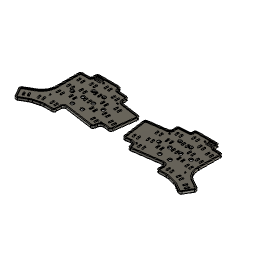
MUSUBI_V2_CASE (Autodesk Fusion 360 design; units mm, degrees)
Autodesk Fusion 360 part; units mm, degrees
note: some values were not read from the file. Set by a fixed rule: which sketch regions a step uses.
sketch "WIP_rev2_case" plane through (0, 0, 0) normal (0, 0, 1) x (1, 0, 0)
  line L0 (119.3956, 43.1697) -> (120.5503, 41.1697)
  line L1 (12.5668, 44.6925) -> (7.0696, 83.8079)
  arc A0 (148.5082, 9.578) -> (145.7761, 8.8459) centre (146.7761, 10.578) cw
  arc A1 (104.7713, 110.126) -> (104.7713, 112.726) centre (104.7713, 111.426) ccw
  line L2 (8.7718, 86.0667) -> (41.7893, 90.7069)
  line L3 (96.0593, 110.126) -> (104.7713, 110.126)
  line L4 (87.3832, 39.0506) -> (35.5891, 31.7716)
  circle A2 centre (69.0928, 67.7697) radius 20.55
  arc A3 (35.5891, 31.7716) -> (33.3302, 33.4738) centre (35.3107, 33.7521) cw
  arc A4 (41.7893, 90.7069) -> (46.9396, 97.0671) centre (40.9543, 96.6485) ccw
  arc A5 (46.5363, 102.8343) -> (48.392, 104.969) centre (48.5315, 102.9738) cw
  line L5 (30.8499, 43.0697) -> (33.1593, 43.0697)
  line L6 (93.8874, 109.0668) -> (92.7327, 111.0668)
  line L7 (90.4233, 107.0668) -> (92.7327, 107.0668)
  line L8 (92.7327, 107.0668) -> (93.8874, 109.0668)
  line L9 (145.7761, 8.8459) -> (133.5777, 15.8887)
  arc A6 (14.8256, 42.9903) -> (12.5668, 44.6925) centre (14.5473, 44.9709) cw
  line L10 (120.5503, 45.1697) -> (119.3956, 43.1697)
  line L11 (48.392, 104.969) -> (64.952, 106.127)
  line L12 (68.673, 110.1172) -> (68.673, 112.1248)
  line L13 (45.7503, 91.2697) -> (44.5956, 89.2697)
  line L14 (107.673, 112.1248) -> (107.673, 106.1248)
  line L15 (70.673, 114.1248) -> (105.673, 114.1248)
  arc A7 (156.0261, 26.5995) -> (156.7582, 23.8674) centre (155.0261, 24.8674) cw
  arc A8 (68.673, 112.1248) -> (70.673, 114.1248) centre (70.673, 112.1248) cw
  line L16 (46.9396, 97.0671) -> (46.5363, 102.8343)
  arc A9 (133.5777, 15.8887) -> (127.7892, 18.2864) centre (121.5777, -4.8959) ccw
  arc A10 (107.673, 106.1248) -> (111.673, 102.1248) centre (111.673, 106.1248) ccw
  line L17 (111.673, 102.1248) -> (124.173, 102.1248)
  arc A11 (96.0593, 105.5236) -> (96.0593, 108.1236) centre (96.0593, 106.8236) cw
  arc A12 (126.173, 60.001) -> (140.173, 35.7523) centre (154.173, 60.001) ccw
  arc A13 (124.173, 102.1248) -> (126.173, 100.1248) centre (124.173, 100.1248) cw
  line L18 (156.7582, 23.8674) -> (148.5082, 9.578)
  circle A14 centre (32.0046, 45.0697) radius 1.3
  line L19 (89.2686, 109.0668) -> (90.4233, 107.0668)
  arc A15 (32.7737, 37.4339) -> (23.7383, 44.2427) centre (24.8515, 36.3206) ccw
  circle A16 centre (106.9188, 67.9606) radius 3.2
  arc A17 (104.7713, 108.1236) -> (104.7713, 105.5236) centre (104.7713, 106.8236) cw
  line L20 (122.8597, 41.1697) -> (124.0144, 43.1697)
  line L21 (33.1593, 47.0697) -> (30.8499, 47.0697)
  circle A18 centre (50.0544, 67.1169) radius 3.2
  arc A19 (7.0696, 83.8079) -> (8.7718, 86.0667) centre (9.0501, 84.0862) cw
  circle A20 centre (91.578, 109.0668) radius 1.3
  arc A21 (105.673, 114.1248) -> (107.673, 112.1248) centre (105.673, 112.1248) cw
  circle A22 centre (69.7456, 48.7314) radius 3.2
  arc A23 (96.2183, 22.1248) -> (94.2183, 24.1248) centre (96.2183, 24.1248) cw
  line L22 (126.173, 100.1248) -> (126.173, 60.001)
  line L23 (49.2144, 89.2697) -> (48.0597, 91.2697)
  line L24 (92.7327, 111.0668) -> (90.4233, 111.0668)
  circle A24 centre (68.8188, 67.9849) radius 3.2
  line L25 (122.8597, 45.1697) -> (120.5503, 45.1697)
  line L26 (90.4233, 111.0668) -> (89.2686, 109.0668)
  line L27 (104.7713, 112.726) -> (96.0593, 112.726)
  line L28 (34.314, 45.0697) -> (33.1593, 47.0697)
  line L29 (45.7503, 87.2697) -> (48.0597, 87.2697)
  arc A25 (94.2183, 33.109) -> (87.3832, 39.0506) centre (88.2183, 33.109) ccw
  line L30 (23.7383, 44.2427) -> (14.8256, 42.9903)
  line L31 (29.6952, 45.0697) -> (30.8499, 43.0697)
  line L32 (48.0597, 91.2697) -> (45.7503, 91.2697)
  circle A26 centre (87.8567, 48.9227) radius 3.2
  line L33 (33.1593, 43.0697) -> (34.314, 45.0697)
  circle A27 centre (88.1311, 68.4225) radius 3.2
  circle A28 centre (87.881, 87.0227) radius 3.2
  line L34 (30.8499, 47.0697) -> (29.6952, 45.0697)
  line L35 (48.0597, 87.2697) -> (49.2144, 89.2697)
  line L36 (33.3302, 33.4738) -> (32.7737, 37.4339)
  line L37 (110.304, 22.1248) -> (96.2183, 22.1248)
  line L38 (120.5503, 41.1697) -> (122.8597, 41.1697)
  circle A29 centre (46.905, 89.2697) radius 1.3
  circle A30 centre (121.705, 43.1697) radius 1.3
  circle A31 centre (87.8688, 67.9727) radius 20.55
  circle A32 centre (68.44, 86.8081) radius 3.2
  line L39 (96.0593, 108.1236) -> (104.7713, 108.1236)
  line L40 (104.7713, 105.5236) -> (96.0593, 105.5236)
  arc A33 (96.0593, 112.726) -> (96.0593, 110.126) centre (96.0593, 111.426) ccw
  arc A34 (64.952, 106.127) -> (68.673, 110.1172) centre (64.673, 110.1172) ccw
  line L41 (140.173, 35.7523) -> (156.0261, 26.5995)
  line L42 (44.5956, 89.2697) -> (45.7503, 87.2697)
  line L43 (124.0144, 43.1697) -> (122.8597, 45.1697)
  arc A35 (116.5155, 21.3071) -> (110.304, 22.1248) centre (110.304, -1.8752) ccw
  line L44 (127.7892, 18.2864) -> (116.5155, 21.3071)
  line L45 (87.6616, 37.0701) -> (35.8674, 29.791)
  arc A36 (30.7931, 37.1556) -> (24.0166, 42.2622) centre (24.8515, 36.3206) ccw
  arc A37 (35.8674, 29.791) -> (31.3497, 33.1954) centre (35.3107, 33.7521) cw
  line L46 (94.2183, 24.1248) -> (94.2183, 33.109)
  arc A38 (92.2183, 33.109) -> (87.6616, 37.0701) centre (88.2183, 33.109) ccw
  line L47 (31.3497, 33.1954) -> (30.7931, 37.1556)
  line L48 (24.0166, 42.2622) -> (15.1039, 41.0098)
  arc A39 (15.1039, 41.0098) -> (10.5862, 44.4142) centre (14.5473, 44.9709) cw
  arc A40 (105.673, 116.1248) -> (109.673, 112.1248) centre (105.673, 112.1248) cw
  arc A41 (64.8125, 108.1221) -> (66.673, 110.1172) centre (64.673, 110.1172) ccw
  line L49 (44.9445, 96.9276) -> (44.5412, 102.6948)
  line L50 (109.673, 112.1248) -> (109.673, 106.1248)
  line L51 (10.5862, 44.4142) -> (5.0891, 83.5295)
  line L52 (8.4935, 88.0473) -> (41.5109, 92.6875)
  arc A42 (44.5412, 102.6948) -> (48.2524, 106.9641) centre (48.5315, 102.9738) cw
  arc A43 (66.673, 112.1248) -> (70.673, 116.1248) centre (70.673, 112.1248) cw
  line L53 (66.673, 110.1172) -> (66.673, 112.1248)
  line L54 (48.2524, 106.9641) -> (64.8125, 108.1221)
  line L55 (70.673, 116.1248) -> (105.673, 116.1248)
  arc A44 (41.5109, 92.6875) -> (44.9445, 96.9276) centre (40.9543, 96.6485) ccw
  arc A45 (5.0891, 83.5295) -> (8.4935, 88.0473) centre (9.0501, 84.0862) cw
  arc A46 (115.9979, 19.3752) -> (110.304, 20.1248) centre (110.304, -1.8752) ccw
  line L56 (127.2716, 16.3545) -> (115.9979, 19.3752)
  line L57 (141.173, 37.4843) -> (157.0261, 28.3315)
  arc A47 (132.5777, 14.1567) -> (127.2716, 16.3545) centre (121.5777, -4.8959) ccw
  arc A48 (128.173, 60.001) -> (141.173, 37.4843) centre (154.173, 60.001) ccw
  line L58 (144.7761, 7.1139) -> (132.5777, 14.1567)
  line L59 (158.4902, 22.8674) -> (150.2402, 8.578)
  arc A49 (96.2183, 20.1248) -> (92.2183, 24.1248) centre (96.2183, 24.1248) cw
  line L60 (110.304, 20.1248) -> (96.2183, 20.1248)
  arc A50 (124.173, 104.1248) -> (128.173, 100.1248) centre (124.173, 100.1248) cw
  arc A51 (109.673, 106.1248) -> (111.673, 104.1248) centre (111.673, 106.1248) ccw
  line L61 (92.2183, 24.1248) -> (92.2183, 33.109)
  line L62 (111.673, 104.1248) -> (124.173, 104.1248)
  arc A52 (157.0261, 28.3315) -> (158.4902, 22.8674) centre (155.0261, 24.8674) cw
  line L63 (128.173, 100.1248) -> (128.173, 60.001)
  arc A53 (150.2402, 8.578) -> (144.7761, 7.1139) centre (146.7761, 10.578) cw
  line L64 (123.5064, 33.035) -> (122.2398, 28.302)
  arc A54 (130.1076, 31.2655) -> (127.5989, 31.9385) centre (128.8534, 31.6024) ccw
  line L65 (130.1078, 31.2662) -> (128.8381, 26.5332)
  arc A55 (143.3657, 25.4077) -> (141.1158, 26.7058) centre (142.2409, 26.0571) ccw
  line L66 (127.5989, 31.9385) -> (126.3293, 27.2062)
  arc A56 (126.3293, 27.2062) -> (128.8381, 26.5332) centre (127.5837, 26.8697) ccw
  arc A57 (138.6673, 22.4618) -> (140.9172, 21.1638) centre (139.7922, 21.8128) ccw
  line L67 (141.1162, 26.7065) -> (138.6673, 22.4618)
  line L68 (149.2844, 21.9906) -> (146.8328, 17.7474)
  line L69 (143.3657, 25.4077) -> (140.9172, 21.1638)
  line L70 (147.0349, 23.2893) -> (144.5838, 19.0469)
  arc A58 (144.5838, 19.0469) -> (146.8328, 17.7474) centre (145.7083, 18.3971) ccw
  arc A59 (149.284, 21.9899) -> (147.0349, 23.2893) centre (148.1596, 22.6399) ccw
  arc A60 (99.7539, 30.3621) -> (102.3513, 30.3629) centre (101.0526, 30.3625) ccw
  line L71 (99.7524, 35.2625) -> (99.7539, 30.3621)
  arc A61 (102.3498, 35.2625) -> (99.7524, 35.2617) centre (101.0511, 35.2625) ccw
  arc A62 (106.5852, 30.3629) -> (109.1827, 30.3621) centre (107.8839, 30.3625) ccw
  arc A63 (109.1842, 35.2617) -> (106.5867, 35.2625) centre (107.8854, 35.2625) ccw
  line L72 (102.3498, 35.2625) -> (102.3513, 30.3629)
  line L73 (120.6389, 57.7625) -> (120.6374, 52.8621)
  arc A64 (113.8046, 76.2625) -> (111.2071, 76.2617) centre (112.5058, 76.2625) ccw
  arc A65 (120.6389, 76.2617) -> (118.0414, 76.2625) centre (119.3402, 76.2625) ccw
  line L74 (120.6389, 94.7625) -> (120.6374, 89.8621)
  line L75 (118.0414, 76.2625) -> (118.0399, 71.3629)
  arc A66 (113.8046, 94.7625) -> (111.2071, 94.7617) centre (112.5058, 94.7625) ccw
  line L76 (120.6389, 76.2625) -> (120.6374, 71.3621)
  arc A67 (120.6389, 57.7617) -> (118.0414, 57.7625) centre (119.3402, 57.7625) ccw
  line L77 (111.2071, 94.7625) -> (111.2086, 89.8621)
  arc A68 (111.2086, 52.8621) -> (113.8061, 52.8629) centre (112.5073, 52.8625) ccw
  line L78 (113.8046, 94.7625) -> (113.8061, 89.8629)
  arc A69 (95.3046, 61.7625) -> (92.7071, 61.7617) centre (94.0058, 61.7625) ccw
  line L79 (118.0414, 94.7625) -> (118.0399, 89.8629)
  line L80 (109.1842, 35.2625) -> (109.1827, 30.3621)
  line L81 (113.8046, 57.7625) -> (113.8061, 52.8629)
  line L82 (111.2071, 76.2625) -> (111.2086, 71.3621)
  arc A70 (113.8046, 57.7625) -> (111.2071, 57.7617) centre (112.5058, 57.7625) ccw
  arc A71 (118.0399, 52.8629) -> (120.6374, 52.8621) centre (119.3387, 52.8625) ccw
  arc A72 (111.2086, 89.8621) -> (113.8061, 89.8629) centre (112.5073, 89.8625) ccw
  line L83 (95.3046, 61.7625) -> (95.3061, 56.8629)
  line L84 (106.5867, 35.2625) -> (106.5852, 30.3629)
  arc A73 (102.1389, 61.7617) -> (99.5414, 61.7625) centre (100.8402, 61.7625) ccw
  arc A74 (118.0399, 71.3629) -> (120.6374, 71.3621) centre (119.3387, 71.3625) ccw
  line L85 (113.8046, 76.2625) -> (113.8061, 71.3629)
  arc A75 (102.1389, 80.2617) -> (99.5414, 80.2625) centre (100.8402, 80.2625) ccw
  line L86 (92.7071, 61.7625) -> (92.7086, 56.8621)
  arc A76 (95.3046, 80.2625) -> (92.7071, 80.2617) centre (94.0058, 80.2625) ccw
  arc A77 (99.5399, 56.8629) -> (102.1374, 56.8621) centre (100.8387, 56.8625) ccw
  line L87 (95.3046, 80.2625) -> (95.3061, 75.3629)
  arc A78 (92.7086, 75.3621) -> (95.3061, 75.3629) centre (94.0073, 75.3625) ccw
  arc A79 (120.6389, 94.7617) -> (118.0414, 94.7625) centre (119.3402, 94.7625) ccw
  arc A80 (111.2086, 71.3621) -> (113.8061, 71.3629) centre (112.5073, 71.3625) ccw
  line L88 (102.1389, 61.7625) -> (102.1374, 56.8621)
  arc A81 (118.0399, 89.8629) -> (120.6374, 89.8621) centre (119.3387, 89.8625) ccw
  line L89 (99.5414, 61.7625) -> (99.5399, 56.8629)
  line L90 (111.2071, 57.7625) -> (111.2086, 52.8621)
  line L91 (118.0414, 57.7625) -> (118.0399, 52.8629)
  arc A82 (92.7086, 56.8621) -> (95.3061, 56.8629) centre (94.0073, 56.8625) ccw
  line L92 (92.7071, 80.2625) -> (92.7086, 75.3621)
  arc A83 (92.7086, 93.8621) -> (95.3061, 93.8629) centre (94.0073, 93.8625) ccw
  arc A84 (99.5399, 93.8629) -> (102.1374, 93.8621) centre (100.8387, 93.8625) ccw
  arc A85 (95.3046, 98.7625) -> (92.7071, 98.7617) centre (94.0058, 98.7625) ccw
  line L93 (95.3046, 98.7625) -> (95.3061, 93.8629)
  arc A86 (76.8046, 106.7625) -> (74.2071, 106.7617) centre (75.5058, 106.7625) ccw
  line L94 (102.1389, 80.2625) -> (102.1374, 75.3621)
  arc A87 (99.5399, 75.3629) -> (102.1374, 75.3621) centre (100.8387, 75.3625) ccw
  arc A88 (74.2086, 101.8621) -> (76.8061, 101.8629) centre (75.5073, 101.8625) ccw
  line L95 (102.1389, 98.7625) -> (102.1374, 93.8621)
  line L96 (99.5414, 98.7625) -> (99.5399, 93.8629)
  line L97 (99.5414, 80.2625) -> (99.5399, 75.3629)
  line L98 (92.7071, 98.7625) -> (92.7086, 93.8621)
  arc A89 (102.1389, 98.7617) -> (99.5414, 98.7625) centre (100.8402, 98.7625) ccw
  arc A90 (81.0399, 83.3629) -> (83.6374, 83.3621) centre (82.3387, 83.3625) ccw
  line L99 (55.0222, 98.0523) -> (55.3655, 93.1647)
  arc A91 (83.6389, 88.2617) -> (81.0414, 88.2625) centre (82.3402, 88.2625) ccw
  arc A92 (76.8046, 69.7625) -> (74.2071, 69.7617) centre (75.5058, 69.7625) ccw
  line L100 (74.2071, 88.2625) -> (74.2086, 83.3621)
  arc A93 (46.6007, 46.5841) -> (44.0284, 46.2234) centre (45.3145, 46.4041) ccw
  line L101 (83.6389, 106.7625) -> (83.6374, 101.8621)
  line L102 (81.0414, 106.7625) -> (81.0399, 101.8629)
  arc A94 (57.6032, 61.1424) -> (55.0121, 60.9605) centre (56.3076, 61.0518) ccw
  arc A95 (74.2086, 64.8621) -> (76.8061, 64.8629) centre (75.5073, 64.8625) ccw
  line L103 (83.6389, 88.2625) -> (83.6374, 83.3621)
  arc A96 (64.4209, 61.6184) -> (61.8297, 61.438) centre (63.1253, 61.5286) ccw
  line L104 (76.8046, 69.7625) -> (76.8061, 64.8629)
  line L105 (59.2487, 98.3479) -> (59.589, 93.4601)
  line L106 (64.4209, 61.6192) -> (64.7612, 56.7306)
  arc A97 (55.0222, 98.0523) -> (52.4311, 97.8703) centre (53.7266, 97.9617) ccw
  line L107 (61.8399, 98.5291) -> (62.1802, 93.6405)
  line L108 (74.2071, 106.7625) -> (74.2086, 101.8621)
  line L109 (81.0414, 69.7625) -> (81.0399, 64.8629)
  arc A98 (37.944, 40.4197) -> (40.5161, 40.782) centre (39.2301, 40.6008) ccw
  arc A99 (81.0399, 64.8629) -> (83.6374, 64.8621) centre (82.3387, 64.8625) ccw
  line L110 (52.431, 97.8711) -> (52.7744, 92.9827)
  arc A100 (61.8399, 98.5283) -> (59.2487, 98.3479) centre (60.5443, 98.4385) ccw
  arc A101 (63.1304, 80.0733) -> (60.5392, 79.8929) centre (61.8348, 79.9835) ccw
  line L111 (83.6389, 69.7625) -> (83.6374, 64.8621)
  arc A102 (74.2086, 83.3621) -> (76.8061, 83.3629) centre (75.5073, 83.3625) ccw
  line L112 (63.1304, 80.0741) -> (63.4707, 75.1855)
  line L113 (60.5392, 79.8929) -> (60.8795, 75.0051)
  line L114 (74.2071, 69.7625) -> (74.2086, 64.8621)
  arc A103 (83.6389, 106.7617) -> (81.0414, 106.7625) centre (82.3402, 106.7625) ccw
  arc A104 (39.8328, 45.6337) -> (37.2607, 45.2714) centre (38.5467, 45.453) ccw
  line L115 (76.8046, 88.2625) -> (76.8061, 83.3629)
  arc A105 (60.8795, 75.0051) -> (63.4707, 75.1855) centre (62.1751, 75.0953) ccw
  line L116 (56.3127, 79.5974) -> (56.656, 74.7098)
  arc A106 (52.7744, 92.9827) -> (55.3655, 93.1647) centre (54.0699, 93.0737) ccw
  line L117 (81.0414, 88.2625) -> (81.0399, 83.3629)
  arc A107 (83.6389, 69.7617) -> (81.0414, 69.7625) centre (82.3402, 69.7625) ccw
  arc A108 (55.3554, 56.0729) -> (57.9465, 56.2549) centre (56.6509, 56.1639) ccw
  line L118 (57.6032, 61.1424) -> (57.9465, 56.2549)
  arc A109 (81.0399, 101.8629) -> (83.6374, 101.8621) centre (82.3387, 101.8625) ccw
  line L119 (76.8046, 106.7625) -> (76.8061, 101.8629)
  line L120 (55.0121, 60.9612) -> (55.3554, 56.0729)
  arc A110 (76.8046, 88.2625) -> (74.2071, 88.2617) centre (75.5058, 88.2625) ccw
  arc A111 (54.0649, 74.5278) -> (56.656, 74.7098) centre (55.3604, 74.6188) ccw
  line L121 (37.2606, 45.2722) -> (37.944, 40.4197)
  arc A112 (56.3127, 79.5974) -> (53.7216, 79.4154) centre (55.0171, 79.5068) ccw
  arc A113 (62.17, 56.5502) -> (64.7612, 56.7306) centre (63.4656, 56.6404) ccw
  arc A114 (59.589, 93.4601) -> (62.1802, 93.6405) centre (60.8846, 93.5503) ccw
  line L122 (39.8328, 45.6337) -> (40.5161, 40.782)
  line L123 (61.8297, 61.438) -> (62.17, 56.5502)
  line L124 (53.7215, 79.4162) -> (54.0649, 74.5278)
  line L125 (46.6006, 46.5848) -> (47.2811, 41.7319)
  arc A115 (44.7088, 41.3712) -> (47.2811, 41.7319) centre (45.9949, 41.5515) ccw
  arc A116 (32.7947, 77.0596) -> (35.3668, 77.4219) centre (34.0807, 77.2408) ccw
  line L126 (34.6834, 82.2736) -> (35.3668, 77.4219)
  line L127 (37.2581, 63.9537) -> (37.9414, 59.1019)
  arc A117 (44.026, 64.904) -> (41.4537, 64.5433) centre (42.7398, 64.7241) ccw
  arc A118 (17.1805, 51.6392) -> (19.7526, 52.0015) centre (18.4666, 51.8204) ccw
  line L128 (41.4512, 83.2248) -> (42.1317, 78.3718)
  arc A119 (34.6834, 82.2736) -> (32.1113, 81.9114) centre (33.3973, 82.0929) ccw
  arc A120 (19.0692, 56.8532) -> (16.4971, 56.491) centre (17.7831, 56.6725) ccw
  arc A121 (37.2581, 63.9537) -> (34.686, 63.5914) centre (35.972, 63.7729) ccw
  line L129 (34.6859, 63.5922) -> (35.3693, 58.7397)
  arc A122 (39.5594, 78.0111) -> (42.1317, 78.3718) centre (40.8456, 78.1915) ccw
  line L130 (38.879, 82.8633) -> (39.5594, 78.0111)
  arc A123 (41.4513, 83.224) -> (38.879, 82.8633) centre (40.1651, 83.044) ccw
  line L131 (44.0259, 64.9048) -> (44.7064, 60.0519)
  arc A124 (42.1341, 59.6912) -> (44.7064, 60.0519) centre (43.4202, 59.8715) ccw
  line L132 (32.1112, 81.9121) -> (32.7947, 77.0596)
  line L133 (44.0284, 46.2234) -> (44.7088, 41.3712)
  line L134 (41.4537, 64.5433) -> (42.1341, 59.6912)
  arc A125 (35.3693, 58.7397) -> (37.9414, 59.1019) centre (36.6554, 58.9208) ccw
  line L135 (16.497, 56.4917) -> (17.1805, 51.6392)
  line L136 (19.0692, 56.8532) -> (19.7526, 52.0015)
  arc A126 (25.8372, 57.8036) -> (23.2648, 57.4429) centre (24.5509, 57.6236) ccw
  arc A127 (23.9452, 52.5907) -> (26.5175, 52.9514) centre (25.2314, 52.7711) ccw
  arc A128 (123.5064, 33.035) -> (120.9972, 33.7065) centre (122.2519, 33.3712) ccw
  line L137 (25.837, 57.8044) -> (26.5175, 52.9514)
  line L138 (23.2648, 57.4429) -> (23.9452, 52.5907)
  line L139 (120.9974, 33.7073) -> (119.7306, 28.9735)
  arc A129 (119.7306, 28.9735) -> (122.2398, 28.302) centre (120.9852, 28.6377) ccw
extrude "Extrude1" add sketch "WIP_rev2_case" along normal blind 4.6 contours L0 L10 L20 L25 L38 L43 | L1 A0 L2 L4 A3 A4 A5 L9 A6 L11 L12 L14 L15 A7 A8 L16 A9 A10 L17 A12 A13 L18 A15 A19 A21 A23 L22 A25 L30 L36 L37 A34 L41 A35 L44 L46 | A1 L3 L27 A33 | A2 A27 | A2 A27 | A2 A24 A27 A31 A90 A102 L115 L117 | A2 A16 A26 A27 A28 A31 A90 L103 | A2 A90 L117 | A2 A31 A90 L103 L117 | A2 A18 A22 A24 A31 A32 L100 A102 | A2 A31 L117 | A2 A22 | A2 A22 | A24 A31 | A24 A31 | A26 A31 | A26 A31 | A2 A31 L115 | A31 A91 L103 L117 | A2 A31 L100 A102 L115 | A2 L100 L115 A110 | A31 A102 L115 | A28 A31 | A28 A31 | A2 A18 | A2 A18 | A16 A31 | A16 A31 | A2 A32 | A2 A32 | L5 L21 L28 L31 L33 L34 | L6 L7 L8 L19 L24 L26 | L13 L23 L29 L32 L35 L42 | A11 A17 L39 L40 | A14 | A20 | A29 | A30 | L45 A36 A37 A38 L47 L48 A39 A40 A41 L49 L50 L51 L52 A42 A43 L53 L54 L55 A44 A45 A46 L56 L57 A47 A48 L58 L59 A49 L60 A50 A51 L61 L62 A52 L63 A53 | L64 A128 L139 A129 | A54 L65 L66 A56 | A55 A57 L67 L69 | L68 L70 A58 A59 | A60 L71 A61 L72 | A62 A63 L80 L84 | L73 A67 A71 L91 | A64 L82 L85 A80 | A65 L75 L76 A74 | L74 L79 A79 A81 | A66 L77 L78 A72 | A68 L81 A70 L90 | A69 L83 L86 A82 | A73 A77 L88 L89 | A75 L94 A87 L97 | A76 L87 A78 L92 | A83 A85 L93 L98 | A84 L95 L96 A89 | A86 A88 L108 L119 | L99 A97 L110 A106 | A92 A95 L104 L114 | A93 L125 A115 L133 | L101 L102 A103 A109 | A94 A108 L118 L120 | A96 L106 A113 L123 | L105 L107 A100 A114 | L109 A99 L111 A107 | A98 A104 L121 L122 | A101 L112 L113 A105 | L116 A111 A112 L124 | A116 L126 A119 L132 | L127 A121 L129 A125 | A117 L131 A124 L134 | A118 A120 L135 L136 | L128 A122 L130 A123 | A126 A127 L137 L138 makes body 1
sketch "Sketch2" plane through (0, 0, 4.6) normal (0, 0, 1) x (-1, 0, 0)
  line L0 (-150.2402, -8.578) -> (-158.4902, -22.8674)
  arc A0 (-158.4902, -22.8674) -> (-157.0261, -28.3315) centre (-155.0261, -24.8674) ccw
  line L1 (-157.0261, -28.3315) -> (-141.173, -37.4843)
  arc A1 (-128.173, -60.001) -> (-141.173, -37.4843) centre (-154.173, -60.001) ccw
  line L2 (-128.173, -60.001) -> (-128.173, -100.1248)
  arc A2 (-128.173, -100.1248) -> (-124.173, -104.1248) centre (-124.173, -100.1248) ccw
  line L3 (-124.173, -104.1248) -> (-111.673, -104.1248)
  arc A3 (-109.673, -106.1248) -> (-111.673, -104.1248) centre (-111.673, -106.1248) ccw
  line L4 (-109.673, -106.1248) -> (-109.673, -112.1248)
  arc A4 (-109.673, -112.1248) -> (-105.673, -116.1248) centre (-105.673, -112.1248) ccw
  line L5 (-105.673, -116.1248) -> (-70.673, -116.1248)
  arc A5 (-70.673, -116.1248) -> (-66.673, -112.1248) centre (-70.673, -112.1248) ccw
  line L6 (-66.673, -112.1248) -> (-66.673, -110.1172)
  arc A6 (-64.8125, -108.1221) -> (-66.673, -110.1172) centre (-64.673, -110.1172) ccw
  line L7 (-64.8125, -108.1221) -> (-48.2524, -106.9641)
  arc A7 (-48.2524, -106.9641) -> (-44.5412, -102.6948) centre (-48.5315, -102.9738) ccw
  line L8 (-44.5412, -102.6948) -> (-44.9445, -96.9276)
  arc A8 (-41.5109, -92.6875) -> (-44.9445, -96.9276) centre (-40.9543, -96.6485) ccw
  line L9 (-41.5109, -92.6875) -> (-8.4935, -88.0473)
  arc A9 (-8.4935, -88.0473) -> (-5.0891, -83.5295) centre (-9.0501, -84.0862) ccw
  line L10 (-5.0891, -83.5295) -> (-10.5862, -44.4142)
  arc A10 (-10.5862, -44.4142) -> (-15.1039, -41.0098) centre (-14.5473, -44.9709) ccw
  line L11 (-15.1039, -41.0098) -> (-24.0166, -42.2622)
  arc A11 (-30.7931, -37.1556) -> (-24.0166, -42.2622) centre (-24.8515, -36.3206) ccw
  line L12 (-30.7931, -37.1556) -> (-31.3497, -33.1954)
  arc A12 (-31.3497, -33.1954) -> (-35.8674, -29.791) centre (-35.3107, -33.7521) ccw
  line L13 (-35.8674, -29.791) -> (-87.6616, -37.0701)
  arc A13 (-92.2183, -33.109) -> (-87.6616, -37.0701) centre (-88.2183, -33.109) ccw
  line L14 (-92.2183, -33.109) -> (-92.2183, -24.1248)
  arc A14 (-92.2183, -24.1248) -> (-96.2183, -20.1248) centre (-96.2183, -24.1248) ccw
  line L15 (-96.2183, -20.1248) -> (-110.304, -20.1248)
  arc A15 (-115.9979, -19.3752) -> (-110.304, -20.1248) centre (-110.304, 1.8752) ccw
  line L16 (-115.9979, -19.3752) -> (-127.2716, -16.3545)
  arc A16 (-132.5777, -14.1567) -> (-127.2716, -16.3545) centre (-121.5777, 4.8959) ccw
  line L17 (-132.5777, -14.1567) -> (-144.7761, -7.1139)
  arc A17 (-144.7761, -7.1139) -> (-150.2402, -8.578) centre (-146.7761, -10.578) ccw
  arc A18 (-94.2183, -33.109) -> (-87.3832, -39.0506) centre (-88.2183, -33.109) ccw
  line L18 (-35.5891, -31.7716) -> (-87.3832, -39.0506)
  arc A19 (-33.3302, -33.4738) -> (-35.5891, -31.7716) centre (-35.3107, -33.7521) ccw
  line L19 (-32.7737, -37.4339) -> (-33.3302, -33.4738)
  arc A20 (-32.7737, -37.4339) -> (-23.7383, -44.2427) centre (-24.8515, -36.3206) ccw
  line L20 (-14.8256, -42.9903) -> (-23.7383, -44.2427)
  arc A21 (-12.5668, -44.6925) -> (-14.8256, -42.9903) centre (-14.5473, -44.9709) ccw
  line L21 (-7.0696, -83.8079) -> (-12.5668, -44.6925)
  arc A22 (-8.7718, -86.0667) -> (-7.0696, -83.8079) centre (-9.0501, -84.0862) ccw
  line L22 (-41.7893, -90.7069) -> (-8.7718, -86.0667)
  arc A23 (-41.7893, -90.7069) -> (-46.9396, -97.0671) centre (-40.9543, -96.6485) ccw
  line L23 (-46.5363, -102.8343) -> (-46.9396, -97.0671)
  arc A24 (-48.392, -104.969) -> (-46.5363, -102.8343) centre (-48.5315, -102.9738) ccw
  line L24 (-64.952, -106.127) -> (-48.392, -104.969)
  arc A25 (-64.952, -106.127) -> (-68.673, -110.1172) centre (-64.673, -110.1172) ccw
  line L25 (-68.673, -112.1248) -> (-68.673, -110.1172)
  arc A26 (-70.673, -114.1248) -> (-68.673, -112.1248) centre (-70.673, -112.1248) ccw
  line L26 (-105.673, -114.1248) -> (-70.673, -114.1248)
  arc A27 (-107.673, -112.1248) -> (-105.673, -114.1248) centre (-105.673, -112.1248) ccw
  line L27 (-107.673, -106.1248) -> (-107.673, -112.1248)
  arc A28 (-107.673, -106.1248) -> (-111.673, -102.1248) centre (-111.673, -106.1248) ccw
  line L28 (-124.173, -102.1248) -> (-111.673, -102.1248)
  arc A29 (-126.173, -100.1248) -> (-124.173, -102.1248) centre (-124.173, -100.1248) ccw
  line L29 (-126.173, -60.001) -> (-126.173, -100.1248)
  arc A30 (-126.173, -60.001) -> (-140.173, -35.7523) centre (-154.173, -60.001) ccw
  line L30 (-156.0261, -26.5995) -> (-140.173, -35.7523)
  arc A31 (-156.7582, -23.8674) -> (-156.0261, -26.5995) centre (-155.0261, -24.8674) ccw
  line L31 (-148.5082, -9.578) -> (-156.7582, -23.8674)
  arc A32 (-145.7761, -8.8459) -> (-148.5082, -9.578) centre (-146.7761, -10.578) ccw
  line L32 (-133.5777, -15.8887) -> (-145.7761, -8.8459)
  arc A33 (-133.5777, -15.8887) -> (-127.7892, -18.2864) centre (-121.5777, 4.8959) ccw
  line L33 (-116.5155, -21.3071) -> (-127.7892, -18.2864)
  arc A34 (-116.5155, -21.3071) -> (-110.304, -22.1248) centre (-110.304, 1.8752) ccw
  line L34 (-96.2183, -22.1248) -> (-110.304, -22.1248)
  arc A35 (-94.2183, -24.1248) -> (-96.2183, -22.1248) centre (-96.2183, -24.1248) ccw
  line L35 (-94.2183, -33.109) -> (-94.2183, -24.1248)
  dimension "d3" = -2
extrude "Extrude2" cut sketch "Sketch2" against normal blind 1.6 contours A18 L18 A19 L19 A20 L20 A21 L21 A22 L22 A23 L23 A24 L24 A25 L25 A26 L26 A27 L27 A28 L28 A29 L29 A30 L30 A31 L31 A32 L32 A33 L33 A34 L34 A35 L35 bodies 1
extrude "Extrude3" cut sketch "WIP_rev2_case" along normal blind 5 contours A1 L3 L27 A33 | A2 A27 | A2 A27 | A2 A90 L117 | A2 A31 A90 L103 L117 | A2 A22 | A2 A22 | A24 A31 | A24 A31 | A26 A31 | A26 A31 | A31 A91 L103 L117 | A2 A31 L100 A102 L115 | A2 L100 L115 A110 | A31 A102 L115 | A28 A31 | A28 A31 | A2 A18 | A2 A18 | A16 A31 | A16 A31 | A2 A32 | A2 A32 | A11 A17 L39 L40 | A14 | A20 | A29 | A30 | L64 A128 L139 A129 | A54 L65 L66 A56 | A55 A57 L67 L69 | L68 L70 A58 A59 | A60 L71 A61 L72 | A62 A63 L80 L84 | L73 A67 A71 L91 | A64 L82 L85 A80 | A65 L75 L76 A74 | L74 L79 A79 A81 | A66 L77 L78 A72 | A68 L81 A70 L90 | A69 L83 L86 A82 | A73 A77 L88 L89 | A75 L94 A87 L97 | A76 L87 A78 L92 | A83 A85 L93 L98 | A84 L95 L96 A89 | A86 A88 L108 L119 | L99 A97 L110 A106 | A92 A95 L104 L114 | A93 L125 A115 L133 | L101 L102 A103 A109 | A94 A108 L118 L120 | A96 L106 A113 L123 | L105 L107 A100 A114 | L109 A99 L111 A107 | A98 A104 L121 L122 | A101 L112 L113 A105 | L116 A111 A112 L124 | A116 L126 A119 L132 | L127 A121 L129 A125 | A117 L131 A124 L134 | A118 A120 L135 L136 | L128 A122 L130 A123 | A126 A127 L137 L138 bodies 1
extrude "Extrude4" cut sketch "WIP_rev2_case" along normal blind 1.6 contours L0 L10 L20 L25 L38 L43 | L5 L21 L28 L31 L33 L34 | L6 L7 L8 L19 L24 L26 | L13 L23 L29 L32 L35 L42 bodies 1
extrude "Extrude5" cut sketch "WIP_rev2_case" along normal blind 1 contours A2 A24 A27 A31 A90 A102 L115 L117 | A2 A16 A26 A27 A28 A31 A90 L103 | A2 A18 A22 A24 A31 A32 L100 A102 bodies 1
chamfer "Chamfer1" distance 0.75 angle 45 36 edges at (7.8376, 63.9719, 0) (5.8556, 86.4935, 0) (25.0022, 90.3674, 0) (44.0628, 94.1313, 0) (44.7429, 99.8112, 0) (45.5126, 105.5981, 0) (56.5325, 107.5431, 0) (66.1357, 108.7532, 0) (66.673, 111.121, 0) (67.8446, 114.9532, 0) (88.173, 116.1248, 0) (108.5014, 114.9532, 0) (109.673, 109.1248, 0) (110.2588, 104.7106, 0) (117.923, 104.1248, 0) (127.0014, 102.9532, 0) (128.173, 80.0629, 0) (131.6563, 47.001, 0) (149.0996, 32.9079, 0) (158.8898, 25.9027, 0) (154.3652, 15.7227, 0) (147.8114, 6.7143, 0) (138.6769, 10.6353, 0) (129.9967, 15.4295, 0) (121.6347, 17.8649, 0) (113.1755, 19.9366, 0) (103.2611, 20.1248, 0) (93.3898, 21.2964, 0) (92.2183, 28.6169, 0) (90.8425, 36.1278, 0) (61.7645, 33.4306, 0) (32.9035, 30.5576, 0) (31.0714, 35.1755, 0) (28.4625, 41.1123, 0) (19.5603, 41.636, 0) (12.14, 41.7764, 0) on bodies 1
mirror "Mirror1" about plane through (0, 0, 0) normal (1, 0, 0) of bodies 1 makes body 2
